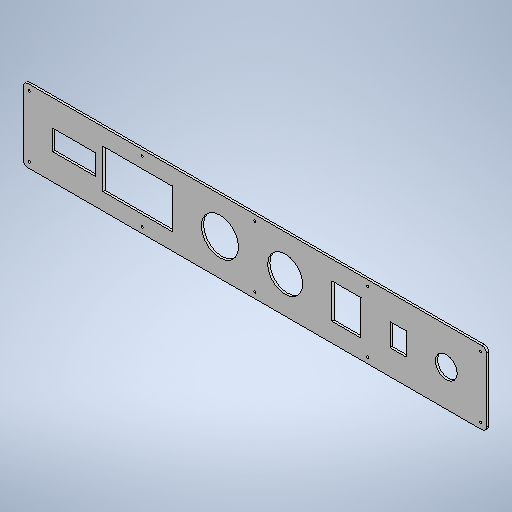
# Autodesk Inventor part: DMF 2.1 Пластина паза маленькая
Saved by Autodesk Inventor 2026.2 (Build 302298010, 298A)
## iProperties
Created: 2024-04-30
Part Number: DMF 2.1 Пластина паза маленькая
Material: Generic
Document SubType Name: Sheet Metal
Designer: pokla
Stock Number: DMF 2.1 Пластина паза маленькая
Density: 1 g/cm^3
Sheet Metal Rule: Default
Sheet Metal Width: 635,000 mm
Sheet Metal Length: 100,000 mm
Sheet Metal Area: 63500,000 mm^2
Appearance: Default
Flat Pattern Width: 63.5 cm
Flat Pattern Length: 10 cm
Flat Pattern Area: 635 cm^2
Author: pokla
Autodesk Inventor part; units mm, degrees
ref_plane "YZ Plane" through (0, 0, 0) normal (1, 0, 0) x (0, 1, 0)
ref_plane "XZ Plane" through (0, 0, 0) normal (0, 1, 0) x (-1, 0, 0)
ref_plane "XY Plane" through (0, 0, 0) normal (0, 0, 1) x (1, 0, 0)
sketch "Sketch1" plane through (0, 0, 0) normal (0, 0, 1) x (1, 0, 0)
  line L0 (-317.5, -50) -> (317.5, -50)
  line L1 (317.5, -50) -> (317.5, 50)
  line L2 (317.5, 50) -> (-317.5, 50)
  line L3 (-317.5, 50) -> (-317.5, -50)
  line L4 (-317.5, -50) -> (317.5, 50) construction
  line L5 (317.5, -50) -> (-317.5, 50) construction
  line L6 (-277.5, 14) -> (-218.5, 14)
  line L7 (-218.5, 14) -> (-218.5, -14)
  line L8 (-218.5, -14) -> (-277.5, -14)
  line L9 (-277.5, -14) -> (-277.5, 14)
  line L10 (-277.5, 14) -> (-218.5, -14) construction
  line L11 (-218.5, 14) -> (-277.5, -14) construction
  line L12 (-208.5, -27) -> (-113.5, -27)
  line L13 (-113.5, -27) -> (-113.5, 27)
  line L14 (-113.5, 27) -> (-208.5, 27)
  line L15 (-208.5, 27) -> (-208.5, -27)
  line L16 (-208.5, -27) -> (-113.5, 27) construction
  line L17 (-113.5, -27) -> (-208.5, 27) construction
  line L18 (-317.5, 0) -> (317.5, 0) construction
  circle A0 centre (-48, 0) radius 25.5
  circle A1 centre (41.5, 0) radius 24
  line L19 (105.5, 24) -> (145.5, 24)
  line L20 (145.5, 24) -> (145.5, -24)
  line L21 (145.5, -24) -> (105.5, -24)
  line L22 (105.5, -24) -> (105.5, 24)
  line L23 (105.5, 24) -> (145.5, -24) construction
  line L24 (145.5, 24) -> (105.5, -24) construction
  line L25 (207.5, -15.5) -> (185.5, -15.5)
  line L26 (185.5, -15.5) -> (185.5, 15.5)
  line L27 (185.5, 15.5) -> (207.5, 15.5)
  line L28 (207.5, 15.5) -> (207.5, -15.5)
  line L29 (207.5, -15.5) -> (185.5, 15.5) construction
  line L30 (185.5, -15.5) -> (207.5, 15.5) construction
  circle A2 centre (262.5, 0) radius 15
  circle A3 centre (0, 42) radius 1.5
  circle A4 centre (154.75, 42) radius 1.5
  circle A5 centre (-154.75, 42) radius 1.5
  circle A6 centre (309.5, 42) radius 1.5
  circle A7 centre (-309.5, 42) radius 1.5
  circle A8 centre (0, -42) radius 1.5
  circle A9 centre (154.75, -42) radius 1.5
  circle A10 centre (-154.75, -42) radius 1.5
  circle A11 centre (309.5, -42) radius 1.5
  circle A12 centre (-309.5, -42) radius 1.5
  point P0 (0, 0)
  point P1 (0, 0)
  point P2 (0, 0)
  point P3 (0, 0)
  point P4 (0, 0)
  point P5 (-248, 0)
  point P6 (-161, 0)
  point P7 (125.5, 0)
  point P8 (196.5, 0)
  point P9 (0, 50)
  dimension "d51" = 635
  dimension "d52" = 100
  dimension "d53" = 59
  dimension "d54" = 28
  dimension "d55" = 95
  dimension "d56" = 54
  dimension "d57" = 51
  dimension "d58" = 48
  dimension "d59" = 40
  dimension "d60" = 48
  dimension "d61" = 22
  dimension "d62" = 31
  dimension "d63" = 30
  dimension "d64" = 40
  dimension "d65" = 55
  dimension "d66" = 55
  dimension "d67" = 64
  dimension "d68" = 89.5
  dimension "d69" = 65.5
  dimension "d70" = 10
  dimension "d71" = 40
  dimension "d84" = 3
  dimension "d85" = 8
  dimension "d88" = 154.75
  measures "d51" distance of L2.end L1.end
  measures "d52" distance of L1.end L0.end
  measures "d53" distance of L7.end L8.end
  measures "d54" distance of L6.end L7.end
  measures "d55" distance of L14.end L13.end
  measures "d56" distance of L13.end L12.end
  measures "d57" diameter of A0
  measures "d58" diameter of A1
  measures "d59" distance of L20.end L21.end
  measures "d60" distance of L19.end L20.end
  measures "d61" distance of L26.end L27.end
  measures "d62" distance of L25.end L26.end
  measures "d63" diameter of A2
  measures "d64" distance between parallel lines of L26 L20
  measures "d65" distance from line of A2.centre L28
  measures "d66" distance from line of A2.centre L1
  measures "d67" distance from line of A1.centre L22
  measures "d68" distance of A1.centre A0.centre
  measures "d69" distance from line of A0.centre L13
  measures "d70" distance between parallel lines of L15 L7
  measures "d71" distance between parallel lines of L3 L9
  measures "d84" diameter of A3
  measures "d85" distance from line of L2 A3.centre
  measures "d88" distance of A3.centre A4.centre
extrude "Plate1" add sketch "Sketch1" along normal blind 3
fillet "Corner Round1" radius 6 4 edges at (-317.5, 50, 1.5) (-317.5, -50, 1.5) (317.5, 50, 1.5) (317.5, -50, 1.5)
equation "\"d66\" = d65"
equation "\"d88\" = -0.5 * d85 + 0.25 * d51"
equation "\"d15\" = Thickness"
equation "\"BendRadius\" = Thickness"
equation "\"BendReliefWidth\" = Thickness"
equation "\"BendReliefDepth\" = 0.5 * Thickness"
equation "\"CornerReliefSize\" = 4 * Thickness"
equation "\"MinimumRemnant\" = 2 * Thickness"
equation "\"TransitionRadius\" = BendRadius"
equation "\"JacobiRadiusSize\" = BendRadius"
equation "\"GapSize\" = Thickness"
equation "\"Thickness\" = 3"
body "Solid1"
